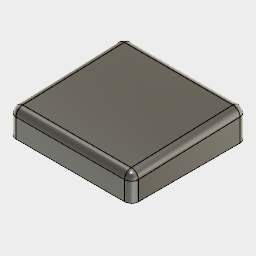
1 (Autodesk Fusion 360 design; units mm, degrees)
Autodesk Fusion 360 part; units mm, degrees
sketch "スケッチ1" plane through (0, 0, 0) normal (0, 0, 1) x (1, 0, 0)
  line L0 (2.5, 2.5) -> (8.2, 2.5)
  line L1 (3, 1) -> (2, 1)
  line L2 (1.9, 1.1) -> (1.9, 3.9)
  line L3 (2, 4) -> (3, 4)
  line L4 (3.1, 3.9) -> (3.1, 1.1)
  line L5 (3.1, 1) -> (1.9, 4) construction
  line L6 (1.9, 1) -> (3.1, 4) construction
  line L7 (8.7, 1) -> (7.7, 1)
  line L8 (7.6, 1.1) -> (7.6, 3.9)
  line L9 (7.7, 4) -> (8.7, 4)
  line L10 (8.8, 3.9) -> (8.8, 1.1)
  line L11 (8.8, 1) -> (7.6, 4) construction
  line L12 (7.6, 1) -> (8.8, 4) construction
  arc A0 (2, 4) -> (1.9, 3.9) centre (2, 3.9) ccw
  arc A1 (3.1, 3.9) -> (3, 4) centre (3, 3.9) ccw
  arc A2 (1.9, 1.1) -> (2, 1) centre (2, 1.1) ccw
  arc A3 (3, 1) -> (3.1, 1.1) centre (3, 1.1) ccw
  arc A4 (7.7, 4) -> (7.6, 3.9) centre (7.7, 3.9) ccw
  arc A5 (8.8, 3.9) -> (8.7, 4) centre (8.7, 3.9) ccw
  arc A6 (7.6, 1.1) -> (7.7, 1) centre (7.7, 1.1) ccw
  arc A7 (8.7, 1) -> (8.8, 1.1) centre (8.7, 1.1) ccw
  point P0 (2.5, 2.5)
  point P1 (8.2, 2.5)
  dimension "d1" = 5.7
  dimension "d2" = 1.2
  dimension "d3" = 3
  dimension "d4" = 3
  dimension "d5" = 1.2
  dimension "d6" = 0.1
  dimension "d7" = 0.1
  dimension "d8" = 0.1
  dimension "d9" = 0.1
  dimension "d10" = 0.1
  dimension "d11" = 0.1
  dimension "d12" = 0.1
  dimension "d13" = 0.1
  measures "d1" distance of P0 L0.end
  measures "d2" distance of L5.end L6.end
  measures "d3" distance of L6.start L5.end
  measures "d4" distance of L12.start L11.end
  measures "d5" distance of L11.end L12.end
  measures "d6" radius of A0
  measures "d7" radius of A1
  measures "d8" radius of A2
  measures "d9" radius of A3
  measures "d10" radius of A4
  measures "d11" radius of A5
  measures "d12" radius of A6
  measures "d13" radius of A7
extrude "押し出し1" add sketch "スケッチ1" along normal blind 3.5 makes body 1 at (1.9, 2.0333, 1.1667) makes body 2 at (7.6, 2.0333, 1.1667)
ref_plane "作業平面1" through (2.5, 2.5, 3.5) normal (0, 0, 1) x (1, 0, 0)
sketch "スケッチ2" plane through (2.5, 2.5, 3.5) normal (0, 0, 1) x (1, 0, 0)
  line L0 (6.3, -1.4) -> (6.3, 1.4)
  line L1 (11.6, -8.25) -> (-5.9, -8.25)
  line L2 (-5.9, -8.25) -> (-5.9, 8.25)
  line L3 (-5.9, 8.25) -> (11.6, 8.25)
  line L4 (11.6, 8.25) -> (11.6, -8.25)
  line L5 (11.6, -8.25) -> (-5.9, 8.25) construction
  line L6 (-5.9, -8.25) -> (11.6, 8.25) construction
  line L7 (2.85, 0) -> (2.85, -1.8)
  line L8 (2.85, 0) -> (2.85, 1.8)
  line L9 (2.85, 0) -> (7.35, 0)
  line L10 (2.85, 0) -> (-1.65, 0)
  line L11 (7.35, 0) -> (7.35, -1.8)
  line L12 (7.35, 0) -> (7.35, 1.8)
  line L13 (-1.65, 0) -> (-1.65, -1.8)
  line L14 (-1.65, 0) -> (-1.65, 1.8)
  line L15 (-1.15, 0) -> (-1.15, -1.8)
  line L16 (-1.15, 0) -> (-1.15, 1.8)
  line L17 (6.85, 0) -> (6.85, -1.8)
  line L18 (6.85, 0) -> (6.85, 1.8)
  line L19 (2.85, 0.25) -> (7.35, 0.25)
  line L20 (2.85, 0.25) -> (-1.65, 0.25)
  line L21 (2.85, -0.25) -> (7.35, -0.25)
  line L22 (2.85, -0.25) -> (-1.65, -0.25)
  line L23 (2.6, 0) -> (2.6, -1.8)
  line L24 (2.6, 0) -> (2.6, 1.8)
  line L25 (3.1, 0) -> (3.1, -1.8)
  line L26 (3.1, 0) -> (3.1, 1.8)
  line L27 (2.6, -1.8) -> (3.1, -1.8)
  line L28 (6.85, -1.8) -> (7.35, -1.8)
  line L29 (6.85, 1.8) -> (7.35, 1.8)
  line L30 (2.6, 1.8) -> (3.1, 1.8)
  line L31 (-1.65, 1.8) -> (-1.15, 1.8)
  line L32 (-1.65, -1.8) -> (-1.15, -1.8)
  point P0 (2.85, 0)
  point P1 (2.85, 0)
  dimension "d17" = 17.5
  dimension "d18" = 16.5
  dimension "d19" = 4.5
  dimension "d20" = 4.5
  dimension "d21" = 0.5
  dimension "d22" = 0.5
  dimension "d23" = 0.25
  dimension "d24" = 0.25
  dimension "d25" = 0.25
  dimension "d26" = 0.25
  measures "d17" distance of L2.end L3.end
  measures "d18" distance of L1.end L2.end
  measures "d19" distance of P1 L9.end
  measures "d20" distance of P1 L10.end
extrude "押し出し2" add sketch "スケッチ2" against normal blind 0.5 contours L0 L9 L21 L25 | L0 L9 L17 L21 | L0 L9 L19 L26 | L0 L9 L18 L19 | L7 L21 L25 L27 | L7 L9 L21 L25 | L11 L17 L21 L28 | L9 L11 L17 L21 | L8 L9 L19 L26 | L9 L12 L18 L19 | L7 L10 L22 L23 | L7 L22 L23 L27 | L8 L19 L26 L30 | L12 L18 L19 L29 | L8 L10 L20 L24 | L10 L15 L22 L23 | L8 L20 L24 L30 | L10 L16 L20 L24 | L10 L13 L15 L22 | L13 L15 L22 L32 | L10 L14 L16 L20 | L14 L16 L20 L31 bodies 1 2
extrude "押し出し3" add sketch "スケッチ2" along normal blind 5 separate body contours L0 L9 L21 L25 | L0 L9 L17 L21 | L0 L9 L19 L26 | L0 L9 L18 L19 | L7 L21 L25 L27 | L7 L9 L21 L25 | L11 L17 L21 L28 | L9 L11 L17 L21 | L8 L9 L19 L26 | L9 L12 L18 L19 | L7 L10 L22 L23 | L7 L22 L23 L27 | L8 L19 L26 L30 | L12 L18 L19 L29 | L8 L10 L20 L24 | L10 L15 L22 L23 | L8 L20 L24 L30 | L10 L16 L20 L24 | L10 L13 L15 L22 | L13 L15 L22 L32 | L10 L14 L16 L20 | L14 L16 L20 L31 | L1 L2 L3 L4 makes body 3
ref_plane "作業平面2" through (-3.4, 2.5, 6) normal (-1, 0, 0) x (0, -1, 0)
sketch "スケッチ3" plane through (-3.4, 2.5, 6) normal (-1, 0, 0) x (0, 1, 0)
  line L0 (1.4, 6) -> (-1.4, 6)
  line L1 (0, 6) -> (0, 0)
  line L2 (12.4924, -0.4362) -> (-12.4924, 0.4362)
  line L3 (8.25, -2.5) -> (-8.25, -2.5)
  line L4 (-8.25, -2.5) -> (-8.25, 2.5)
  line L5 (-8.25, 2.5) -> (8.25, 2.5)
  line L6 (8.25, 2.5) -> (8.25, -2.5)
  line L7 (8.25, -2.5) -> (-8.25, 2.5) construction
  line L8 (-8.25, -2.5) -> (8.25, 2.5) construction
  point P0 (8.25, -2.5)
  dimension "d32" = 6
  measures "d32" distance of L1.start L1.end
extrude "押し出し4" cut sketch "スケッチ3" against normal blind 18 contours L2 L3 L4 L6 bodies 3
sketch "スケッチ4" plane through (2.5, 2.5, 3.5) normal (0, 0, 1) x (1, 0, 0)
  line L0 (10.6, 7.25) -> (-4.9, 7.25)
  line L1 (-4.9, 7.25) -> (-4.9, -7.25)
  line L2 (-4.9, -7.25) -> (10.6, -7.25)
  line L3 (10.6, -7.25) -> (10.6, 7.25)
  line L4 (10.6, 7.25) -> (-4.9, -7.25) construction
  line L5 (-4.9, 7.25) -> (10.6, -7.25) construction
  line L6 (11.6, -8.25) -> (-5.9, -8.25)
  line L7 (-5.9, -8.25) -> (-5.9, 8.25)
  line L8 (-5.9, 8.25) -> (11.6, 8.25)
  line L9 (11.6, 8.25) -> (11.6, -8.25)
  line L10 (11.6, -8.25) -> (-5.9, 8.25) construction
  line L11 (-5.9, -8.25) -> (11.6, 8.25) construction
  point P0 (2.85, 0)
  point P1 (2.85, 0)
  point P2 (2.85, 0)
  point P3 (11.6, -8.25)
  dimension "d35" = 15.5
  dimension "d36" = 14.5
  measures "d35" distance of L1.end L2.end
  measures "d36" distance of L0.end L1.end
extrude "押し出し5" add sketch "スケッチ4" against normal blind 1.5 bodies 3
fillet "フィレット1" radius 1 1 edges at (-3.4, 2.5, 6) on bodies 3
fillet "フィレット2" radius 1 1 edges at (14.1, 2.5, 6) on bodies 3
fillet "フィレット3" radius 1 5 edges at (14.1, -5.75, 3.3556) (13.8071, -5.75, 5.4188) (5.35, -5.75, 5.7119) (-3.1071, -5.75, 5.4188) (-3.4, -5.75, 3.3556) on bodies 3
fillet "フィレット4" radius 1 5 edges at (-3.4, 10.75, 3.6437) (-3.1071, 10.75, 5.995) (5.35, 10.75, 6.2881) (13.8071, 10.75, 5.995) (14.1, 10.75, 3.6437) on bodies 3
fillet "フィレット5" radius 2 4 edges at (13.1, 2.5, 3.5) (5.35, 9.75, 3.5) (-2.4, 2.5, 3.5) (5.35, -4.75, 3.5) on bodies 3
fillet "フィレット6" radius 0.1 8 edges at (8.7707, 3.9707, 0) (8.8, 2.5, 0) (8.7707, 1.0293, 0) (8.2, 1, 0) (7.6293, 1.0293, 0) (7.6, 2.5, 0) (7.6293, 3.9707, 0) (8.2, 4, 0) on bodies 1
fillet "フィレット7" radius 0.1 8 edges at (1.9293, 3.9707, 0) (2.5, 4, 0) (3.0707, 3.9707, 0) (3.1, 2.5, 0) (3.0707, 1.0293, 0) (2.5, 1, 0) (1.9293, 1.0293, 0) (1.9, 2.5, 0) on bodies 1
